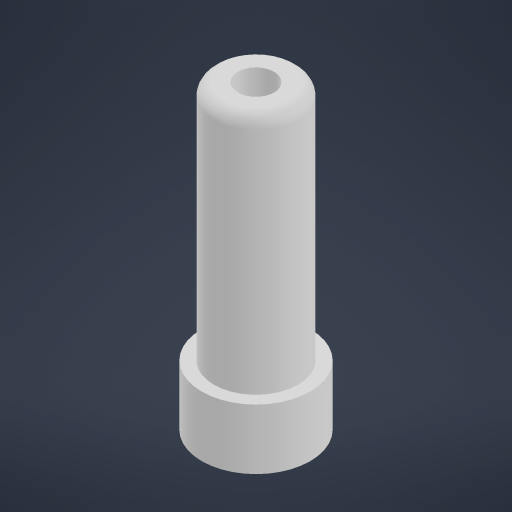
# Autodesk Inventor part: telescopic button bottom
Saved by Autodesk Inventor 2024.1 (Build 281209000, 209)
## iProperties
Created: 2025-01-05
Part Number: telescopic button bottom
Material: Generic
Document SubType Name: Modeling
Designer: Vibhu Iyer
Density: 1 g/cm^3
Appearance: Default
Author: Vibhu Iyer
Autodesk Inventor part; units mm, degrees
ref_plane "YZ Plane" through (0, 0, 0) normal (1, 0, 0) x (0, 1, 0)
ref_plane "XZ Plane" through (0, 0, 0) normal (0, 1, 0) x (-1, 0, 0)
ref_plane "XY Plane" through (0, 0, 0) normal (0, 0, 1) x (1, 0, 0)
sketch "Sketch5" plane through (0, 0, 0) normal (0, 1, 0) x (-1, 0, 0)
  circle A0 centre (0, 0) radius 4.5
  circle A1 centre (0, 0) radius 2.25
  circle A2 centre (0, 0) radius 1.5
  circle A3 centre (0, 0) radius 3.5
  dimension "d43" = 9
  dimension "d44" = 4.5
  dimension "d45" = 3
  dimension "d46" = 7
  constraints: 4 centre point, 3 coincident
  measures "d43" diameter of A0
  measures "d44" diameter of A1
  measures "d45" diameter of A2
  measures "d46" diameter of A3
extrude "Extrusion9" add sketch "Sketch5" along normal blind 5 contours A0 | A3
extrude "Extrusion10" add sketch "Sketch5" along normal blind 20 from surface at 5 contours A1 | A3
fillet "Fillet3" radius 1 1 edges at (3.5, 25, 0)
body "Solid4"
